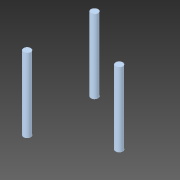
# Autodesk Inventor part: Locate Rig Columns
Saved by Autodesk Inventor 2020.1 (Build 241239000, 239)
## iProperties
Created: 2019-08-27
Part Number: Locate Rig Columns
Material: Steel, Mild
Document SubType Name: Modeling
Designer: Oliver Frolovs
Mass: 5160.42 g
Surface Area: 918.916 cm^2
Volume: 657.378 cm^3
Density: 7.85 g/cm^3
Appearance: Light Steel Blue
Author: Oliver Frolovs
Autodesk Inventor part; units mm, degrees
ref_plane "YZ Plane" through (0, 0, 0) normal (1, 0, 0) x (0, 1, 0)
ref_plane "XZ Plane" through (0, 0, 0) normal (0, 1, 0) x (-1, 0, 0)
ref_plane "XY Plane" through (0, 0, 0) normal (0, 0, 1) x (1, 0, 0)
sketch "Locate Rig Columns" plane through (0, 0, 0) normal (0, 0, 1) x (1, 0, 0)
  circle A0 centre (0, 0) radius 164 construction
  circle A1 centre (0, 164) radius 15
  circle A2 centre (-142.0282, -82) radius 15
  circle A3 centre (142.0282, -82) radius 15
  dimension "d5" = 328
  dimension "d0" = 30
  dimension "d3" = 360
  constraints: 3 centre point, 2 vertical alignment, 1 coincident, 9 other
  measures "d0" diameter of A1
extrude "Extrude Rig Columns" add sketch "Locate Rig Columns" along normal blind 180 and the other way blind 130
equation "\"d5\" = RigColumnsPCD"
equation "\"d0\" = RigColumnsDiameter"
equation "\"RigColumnsPCD\" = 328"
equation "\"RigColumnsDiameter\" = 30"
body "Solid1"
